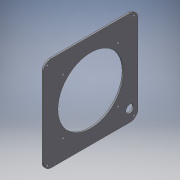
# Autodesk Inventor part: TrayPanelD_120mmAdapter
Saved by Autodesk Inventor 2017 (Build 210142000, 142)
## iProperties
Created: 2019-06-27
Part Number: TrayPanelD_120mmAdapter
Material: Generic
Document SubType Name: Modeling
Designer: DDeGo
Density: 1 g/cm^3
Appearance: Default
Author: DDeGo
Autodesk Inventor part; units mm, degrees
ref_plane "YZ Plane" through (0, 0, 0) normal (1, 0, 0) x (0, 1, 0)
ref_plane "XZ Plane" through (0, 0, 0) normal (0, 1, 0) x (-1, 0, 0)
ref_plane "XY Plane" through (0, 0, 0) normal (0, 0, 1) x (1, 0, 0)
sketch "Sketch1" plane through (0, 0, 0) normal (1, 0, 0) x (0, 1, 0)
  line L0 (15, 0) -> (165, 0)
  line L1 (180, 15) -> (180, 165)
  line L2 (165, 180) -> (15, 180)
  line L3 (0, 165) -> (0, 15)
  line L4 (180, 180) -> (0, 0) construction
  line L5 (30, 30) -> (150, 30) construction
  line L6 (150, 30) -> (150, 150) construction
  line L7 (150, 150) -> (30, 150) construction
  line L8 (30, 150) -> (30, 30) construction
  line L9 (30, 30) -> (150, 150) construction
  line L10 (150, 30) -> (30, 150) construction
  line L11 (37.5, 37.5) -> (142.5, 37.5) construction
  line L12 (142.5, 37.5) -> (142.5, 142.5) construction
  line L13 (142.5, 142.5) -> (37.5, 142.5) construction
  line L14 (37.5, 142.5) -> (37.5, 37.5) construction
  line L15 (37.5, 37.5) -> (142.5, 142.5) construction
  line L16 (142.5, 37.5) -> (37.5, 142.5) construction
  circle A0 centre (142.5, 142.5) radius 2
  circle A1 centre (142.5, 37.5) radius 2
  circle A2 centre (37.5, 37.5) radius 2
  circle A3 centre (37.5, 142.5) radius 2
  circle A4 centre (90, 90) radius 62.5
  arc A5 (180, 165) -> (165, 180) centre (165, 165) ccw
  arc A6 (165, 0) -> (180, 15) centre (165, 15) ccw
  arc A7 (0, 15) -> (15, 0) centre (15, 15) ccw
  arc A8 (15, 180) -> (0, 165) centre (15, 165) ccw
  line L17 (7.5, 7.5) -> (172.5, 7.5) construction
  line L18 (172.5, 7.5) -> (172.5, 172.5) construction
  line L19 (172.5, 172.5) -> (7.5, 172.5) construction
  line L20 (7.5, 172.5) -> (7.5, 7.5) construction
  line L21 (7.5, 7.5) -> (172.5, 172.5) construction
  line L22 (172.5, 7.5) -> (7.5, 172.5) construction
  circle A9 centre (172.5, 172.5) radius 2
  circle A10 centre (172.5, 7.5) radius 2
  circle A11 centre (7.5, 7.5) radius 2
  circle A12 centre (7.5, 172.5) radius 2
  dimension "d0" = 180
  dimension "d1" = 180
  dimension "d2" = 120
  dimension "d3" = 105
  dimension "d4" = 4
  dimension "d5" = 125
  dimension "d6" = 15
  dimension "d9" = 4
  dimension "d10" = 165
  constraints: 46 end point, 13 centre point, 9 coincident, 9 equal radius, 8 parallel, 8 point on circle, 8 tangent, 7 midpoint, 7 point on line, 4 horizontal, 4 perpendicular
  measures "d0" distance between parallel lines of L0 L2
  measures "d1" distance between parallel lines of L3 L1
  measures "d2" distance of L5.end L6.end
  measures "d3" distance of L11.end L12.end
  measures "d4" diameter of A0
  measures "d5" diameter of A4
  measures "d6" radius of A5
  measures "d9" diameter of A9
  measures "d10" distance of L17.end L18.end
extrude "Extrusion1" add sketch "Sketch1" along normal blind 2.75
sketch "Sketch2" plane through (2.75, 0, 0) normal (1, 0, 0) x (0, 0, -1)
  circle A0 centre (-22.5, 164.5) radius 7.5
  circle A1 centre (-7.5, 172.5) radius 2 projected
  point P0 (0, 0)
  dimension "d11" = 15
  dimension "d12" = 15
  dimension "d13" = 8
  constraints: 1 centre point
  measures "d11" diameter of A0
  measures "d12" horizontal distance of A1.centre A0.centre
  measures "d13" vertical distance of A1.centre A0.centre
extrude "Extrusion2" cut sketch "Sketch2" against normal blind 10 contours A0
body "Solid1"
